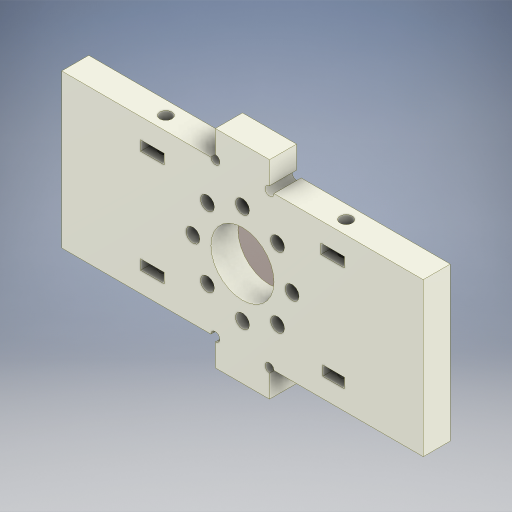
# Autodesk Inventor part: hip joint_body connector
Saved by Autodesk Inventor 2024 (Build 280153000, 153)
## iProperties
Created: 2024-09-03
Part Number: hip joint_body connector
Material: PMMA 플라스틱
Document SubType Name: Modeling
Designer: msi
Density: 1.188 g/cm^3
Appearance: 매끄러움 - 아이보리색
Author: msi
Autodesk Inventor part; units mm, degrees
ref_plane "YZ Plane" through (0, 0, 0) normal (1, 0, 0) x (0, 1, 0)
ref_plane "XZ Plane" through (0, 0, 0) normal (0, 1, 0) x (-1, 0, 0)
ref_plane "XY Plane" through (0, 0, 0) normal (0, 0, 1) x (1, 0, 0)
ref_plane "작업 평면1" through (0, 0, 0) normal (0, 0, 1) x (1, 0, 0)
sketch "스케치1" plane through (0, 0, 0) normal (0, 0, 1) x (1, 0, 0)
  circle A0 centre (-7.7782, -7.7782) radius 1.55 projected
  circle A1 centre (7.7782, -7.7782) radius 1.55 projected
  circle A2 centre (7.7782, 7.7782) radius 1.55 projected
  circle A3 centre (-7.7782, 7.7782) radius 1.55 projected
  circle A4 centre (0, 0) radius 5 projected
  circle A5 centre (0, 0) radius 13.9 projected
  circle A6 centre (0, 11) radius 1.55 projected
  circle A7 centre (11, 0) radius 1.55 projected
  circle A8 centre (0, -11) radius 1.55 projected
  circle A9 centre (-11, 0) radius 1.55 projected
  line L0 (-40.1, -17) -> (40.1, -17)
  line L1 (40.1, -17) -> (40.1, 17)
  line L2 (40.1, 17) -> (-40.1, 17)
  line L3 (-40.1, 17) -> (-40.1, -17)
  line L4 (-40.1, -17) -> (40.1, 17) construction
  line L5 (40.1, -17) -> (-40.1, 17) construction
  circle A10 centre (0, 0) radius 7
  circle A11 centre (0, 11) radius 1.35
  circle A12 centre (-7.7782, 7.7782) radius 1.35
  circle A13 centre (-11, 0) radius 1.35
  circle A14 centre (-7.7782, -7.7782) radius 1.35
  circle A15 centre (0, -11) radius 1.35
  circle A16 centre (7.7782, -7.7782) radius 1.35
  circle A17 centre (11, 0) radius 1.35
  circle A18 centre (7.7782, 7.7782) radius 1.35
  line L6 (6, 17) -> (-6, 17)
  line L7 (-6, 17) -> (-6, 23)
  line L8 (-6, 23) -> (6, 23)
  line L9 (6, 23) -> (6, 17)
  line L10 (6, -17) -> (-6, -17)
  line L11 (-6, -17) -> (-6, -23)
  line L12 (-6, -23) -> (6, -23)
  line L13 (6, -23) -> (6, -17)
  point P0 (0, 0)
  point P1 (0, 0)
  point P2 (0, 0)
  point P3 (0, 0)
  point P4 (0, 0)
  point P5 (0, 0)
  point P6 (0, 0)
  point P7 (0, 0)
  dimension "d0" = 80.2
  dimension "d1" = 34
  dimension "d2" = 2
  dimension "d3" = 2.7
  dimension "d6" = 360
  dimension "d8" = 12
  dimension "d9" = 6
  dimension "d10" = 12
  dimension "d11" = 6
  constraints: 28 end point, 9 centre point, 6 parallel, 3 coincident, 3 horizontal, 3 perpendicular, 2 midpoint, 2 point on line, 23 other
  measures "d0" distance of L2.end L1.end
  measures "d1" distance of L1.end L0.end
  measures "d2" radial gap between concentric circles of A4 A10
  measures "d3" diameter of A11
  measures "d8" distance of L7.end L8.end
  measures "d9" distance of L6.end L7.end
  measures "d10" distance of L12.end L11.end
  measures "d11" distance of L11.end L10.end
extrude "돌출1" add sketch "스케치1" along normal blind 6 contours A5 | L3 L2 L1 L0 | L0 L13 L12 L11 | L7 L8 L9 L2
sketch "스케치3" plane through (-6, 23, 0) normal (0, 1, 0) x (1, 0, 0)
  circle A0 centre (26, -3) radius 1.35
  circle A1 centre (-14, -3) radius 1.35
  point P0 (6, 0)
  dimension "d14" = 2.7
  dimension "d15" = 2.7
  constraints: 2 centre point
  measures "d14" diameter of A0
  measures "d15" diameter of A1
extrude "돌출2" cut sketch "스케치3" against normal blind 100
sketch "스케치4" plane through (0, 0, 6) normal (0, 0, 1) x (1, 0, 0)
  line L0 (22.2, 12.7) -> (17, 10.5) construction
  line L1 (17, 12.7) -> (22.2, 10.5) construction
  line L2 (-22.2, 12.7) -> (-17, 10.5) construction
  line L3 (-17, 12.7) -> (-22.2, 10.5) construction
  line L4 (17.8, -12.7) -> (23, -12.7)
  line L5 (23, -10.5) -> (17.8, -10.5)
  line L6 (17.8, -10.5) -> (17.8, -12.7)
  line L7 (17.8, -12.7) -> (23, -10.5) construction
  line L8 (23, -12.7) -> (17.8, -10.5) construction
  line L9 (-22.2, -12.7) -> (-17, -10.5) construction
  line L10 (-17, -12.7) -> (-22.2, -10.5) construction
  line L11 (18.65, 17) -> (18.65, -17) projected
  line L12 (21.35, 17) -> (21.35, -17) projected
  line L13 (17.4, 10.5) -> (22.6, 10.5)
  line L14 (22.6, 10.5) -> (22.6, 12.7)
  line L15 (22.6, 12.7) -> (17.4, 12.7)
  line L16 (17.4, 12.7) -> (17.4, 10.5)
  line L17 (17.4, 10.5) -> (22.6, 12.7) construction
  line L18 (22.6, 10.5) -> (17.4, 12.7) construction
  line L19 (-22.6, 10.3308) -> (-17.4, 10.3308)
  line L20 (-17.4, 10.3308) -> (-17.4, 12.5308)
  line L21 (-17.4, 12.5308) -> (-22.6, 12.5308)
  line L22 (-22.6, 12.5308) -> (-22.6, 10.3308)
  line L23 (-22.6, 10.3308) -> (-17.4, 12.5308) construction
  line L24 (-17.4, 10.3308) -> (-22.6, 12.5308) construction
  line L25 (22.6, -12.7) -> (22.6, -10.5)
  line L26 (17.4, -12.7) -> (22.6, -10.5) construction
  line L27 (22.6, -12.7) -> (17.4, -10.5) construction
  line L28 (-22.6, -12.531) -> (-17.4, -12.531)
  line L29 (-17.4, -12.531) -> (-17.4, -10.331)
  line L30 (-17.4, -10.331) -> (-22.6, -10.331)
  line L31 (-22.6, -10.331) -> (-22.6, -12.531)
  line L32 (-22.6, -12.531) -> (-17.4, -10.331) construction
  line L33 (-17.4, -12.531) -> (-22.6, -10.331) construction
  point P0 (0, 0)
  point P1 (-19.6, 11.6)
  point P2 (20.4, -11.6)
  point P3 (-19.6, -11.6)
  point P4 (20, 11.6)
  point P5 (-20, 11.4308)
  point P6 (20, -11.6)
  point P7 (-20, -11.431)
  dimension "d18" = 5.2
  dimension "d19" = 2.2
  dimension "d20" = 5.2
  dimension "d21" = 2.2
  dimension "d22" = 5.2
  dimension "d23" = 2.2
  dimension "d24" = 5.2
  dimension "d25" = 2.2
  dimension "d28" = 5.2
  dimension "d29" = 2.2
  dimension "d30" = 5.2
  dimension "d31" = 2.2
  dimension "d32" = 5.2
  dimension "d33" = 2.2
  dimension "d34" = 5.2
  dimension "d35" = 2.2
  constraints: 64 end point, 14 midpoint, 7 parallel, 4 horizontal, 3 perpendicular, 1 point on line
  measures "d18" distance of L1.end L0.end
  measures "d19" distance of L0.end L1.start
  measures "d20" distance of L2.end L3.end
  measures "d21" distance of L3.start L2.end
  measures "d22" distance of L5.end L5.start
  measures "d23" distance of L5.start L4.end
  measures "d24" distance of L10.end L9.end
  measures "d25" distance of L9.end L10.start
  measures "d28" distance of L15.end L14.end
  measures "d29" distance of L14.end L13.end
  measures "d30" distance of L21.end L20.end
  measures "d31" distance of L20.end L19.end
  measures "d32" distance of L27.end L25.end
  measures "d33" distance of L25.end L25.start
  measures "d34" distance of L30.end L29.end
  measures "d35" distance of L29.end L28.end
extrude "돌출4" cut sketch "스케치4" against normal blind 10 contours L6 L5 L11 L4 | L11 L5 L12 L4 | L12 L5 L25 L4 | L13 L16 L15 L11 | L11 L15 L12 L13 | L12 L15 L14 L13 | L22 L21 L20 L19 | L31 L30 L29 L28
sketch "스케치5" plane through (0, 0, 6) normal (0, 0, 1) x (1, 0, 0)
  line L0 (22.6, 10.5) -> (17.4, 10.5) projected
  line L1 (17.4, 10.5) -> (17.4, 12.7) projected
  line L2 (17.4, 12.7) -> (22.6, 12.7) projected
  line L3 (22.6, 12.7) -> (22.6, 10.5) projected
  line L4 (-22.6, -10.331) -> (-17.4, -10.331) projected
  line L5 (-17.4, -10.331) -> (-17.4, -12.531) projected
  line L6 (-17.4, -12.531) -> (-22.6, -12.531) projected
  line L7 (-22.6, -12.531) -> (-22.6, -10.331) projected
  line L8 (17.8, -12.7) -> (17.8, -10.5) projected
  line L9 (17.8, -10.5) -> (22.6, -10.5) projected
  line L10 (22.6, -10.5) -> (22.6, -12.7) projected
  line L11 (22.6, -12.7) -> (17.8, -12.7) projected
  line L12 (-22.6, 12.5308) -> (-17.4, 12.5308) projected
  line L13 (-17.4, 12.5308) -> (-17.4, 10.3308) projected
  line L14 (-17.4, 10.3308) -> (-22.6, 10.3308) projected
  line L15 (-22.6, 10.3308) -> (-22.6, 12.5308) projected
  line L16 (40.1, 17) -> (6, 17) projected
  line L17 (6, 17) -> (6, 23) projected
  line L18 (6, 23) -> (-6, 23) projected
  line L19 (-6, 23) -> (-6, 17) projected
  line L20 (-6, 17) -> (-40.1, 17) projected
  line L21 (-40.1, 17) -> (-40.1, -17) projected
  line L22 (-40.1, -17) -> (-6, -17) projected
  line L23 (-6, -17) -> (-6, -23) projected
  line L24 (-6, -23) -> (6, -23) projected
  line L25 (6, -23) -> (6, -17) projected
  line L26 (6, -17) -> (40.1, -17) projected
  line L27 (40.1, -17) -> (40.1, 17) projected
  circle A0 centre (-7.7782, -7.7782) radius 1.55 projected
  circle A1 centre (7.7782, -7.7782) radius 1.55 projected
  circle A2 centre (7.7782, 7.7782) radius 1.55 projected
  circle A3 centre (-7.7782, 7.7782) radius 1.55 projected
  circle A4 centre (0, 11) radius 1.55 projected
  circle A5 centre (11, 0) radius 1.55 projected
  circle A6 centre (0, -11) radius 1.55 projected
  circle A7 centre (-11, 0) radius 1.55 projected
  circle A8 centre (0, 0) radius 7 projected
  circle A9 centre (6, 17) radius 1
  circle A10 centre (-6, 17) radius 1
  circle A11 centre (6, -17) radius 1
  circle A12 centre (-6, -17) radius 1
  point P0 (0, 0)
  point P1 (-6, 18)
  point P2 (-7, 17)
  point P3 (6, 18)
  point P4 (7, 17)
  point P5 (7, -17)
  point P6 (6, -18)
  dimension "d38" = 2
  dimension "d39" = 2
  dimension "d40" = 2
  dimension "d41" = 2
  constraints: 4 centre point, 4 coincident
  measures "d38" diameter of A9
  measures "d39" diameter of A10
  measures "d40" diameter of A11
  measures "d41" diameter of A12
extrude "돌출5" cut sketch "스케치5" against normal blind 10 contours A9 L17 L16 | L26 L25 A11 | A10 L20 L19 | A12 L22 L23 | L23 L22 A12 picked at (6.5384, 16.6156) picked at (6.5384, -16.6156) picked at (-6.657, 16.9202)
